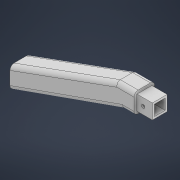
# Autodesk Inventor part: Fahrwerk_rocker_vorne
Saved by Autodesk Inventor 2021 (Build 250183000, 183)
## iProperties
Created: 2020-12-29
Part Number: Fahrwerk_rocker_vorne
Material: Generisch
Document SubType Name: Modeling
Designer: laure
Density: 1 g/cm^3
Appearance: Vorgabe
Author: laure
## iProperties of the stored document _3D-Druck.ipt
Created: 2020-12-30
Part Number: _3D-Druck
Material: Generisch
Document SubType Name: Modeling
Designer: laure
Density: 1 g/cm^3
Appearance: Vorgabe
Author: laure
Autodesk Inventor part; units mm, degrees
ref_plane "YZ Plane" through (0, 0, 0) normal (1, 0, 0) x (0, 1, 0)
ref_plane "XZ Plane" through (0, 0, 0) normal (0, 1, 0) x (-1, 0, 0)
ref_plane "XY Plane" through (0, 0, 0) normal (0, 0, 1) x (1, 0, 0)
sketch "Skizze1" plane through (0, 0, 0) normal (0, 0, 1) x (1, 0, 0)
  line L0 (4.7064, 3.5044) -> (-12.7276, 3.5044)
  line L1 (-12.7276, 3.5044) -> (-116.0937, -34.1178)
  line L2 (4.7064, 3.5044) -> (4.7064, -16.4956)
  line L3 (4.7064, -16.4956) -> (-6.4216, -16.4956)
  line L4 (-6.4216, -16.4956) -> (-116.0937, -55.3341)
  line L5 (-116.0937, -34.1178) -> (-116.0937, -55.4014)
  line L6 (0, 15.2855) -> (0, -67.1826) projected
  line L7 (-140.2538, 0) -> (28.8665, 0) projected
  point P0 (0, 0)
  dimension "d0" = 17.434
  dimension "d1" = 110
  dimension "d4" = 20
  dimension "d5" = 11.128
  dimension "d38" = 4.7065
  dimension "d39" = 16.4956
  dimension "d40" = 20
  dimension "d44" = 160.499
  constraints: 12 end point, 2 vertical, 1 horizontal, 1 parallel, 1 point on line
  measures "d0" distance of L0.start L0.end
  measures "d1" distance of L0.end L1.end
  measures "d4" distance of L0.start L2.end
  measures "d5" distance of L2.end L3.end
  measures "d38" distance from line of point (0, 0) L2
  measures "d39" distance from line of point (0, 0) L3
  measures "d40" angle of L1 L0
  measures "d44" angle of L3 L4
ref_plane "Arbeitsebene2" through (4.7064, -12.4956, -10) normal (1, 0, 0) x (0, 0, -1)
sketch "Skizze3" plane through (4.7064, -12.4956, -10) normal (1, 0, 0) x (0, 0, -1)
  line L0 (-3, -65.9356) -> (-3, 0) projected
  line L1 (-17.2, 13.2) -> (-2.8, 13.2)
  line L2 (-2.8, 13.2) -> (-2.8, -1.2)
  line L3 (-2.8, -1.2) -> (-17.2, -1.2)
  line L4 (-17.2, -1.2) -> (-17.2, 13.2)
  line L5 (-4.8, 11.2) -> (-15.2, 11.2)
  line L6 (-15.2, 11.2) -> (-15.2, 0.8)
  line L7 (-15.2, 0.8) -> (-4.8, 0.8)
  line L8 (-4.8, 0.8) -> (-4.8, 11.2)
  line L9 (-2.8, -1.2) -> (-17.2, -1.2) projected
  line L10 (-17.2, -1.2) -> (-17.2, 13.2) projected
  point P0 (-3, -1.2)
  point P1 (-3, 0)
  dimension "d13" = 14.4
  dimension "d14" = 14.4
  dimension "d15" = 2
  dimension "d31" = 0
  dimension "d32" = 0
  constraints: 16 end point, 4 parallel, 2 perpendicular, 1 horizontal, 3 other
  measures "d13" distance of L2.end L3.end
  measures "d14" distance of L1.end L2.end
  measures "d15" distance between parallel lines of L1 L5
  measures "d31" distance between parallel lines of L9 L3
  measures "d32" distance between parallel lines of L10 L4
extrude "Extrusion2" add sketch "Skizze3" along normal blind 15 and the other way blind 7.5
sketch "Skizze5" plane through (-2.7936, -13.6956, 7.2) normal (0, 0, 1) x (1, 0, 0)
  circle A0 centre (13.5, 7.2) radius 1.6
  line L0 (22.5, 14.4) -> (22.5, 0) projected
  line L1 (0, 0) -> (22.5, 0) projected
  dimension "d29" = 3.2
  dimension "d47" = 7.2
  dimension "d48" = 9
  constraints: 1 centre point
  measures "d29" diameter of A0
  measures "d47" distance from line of L1 A0.centre
  measures "d48" distance from line of L0 A0.centre
extrude "Extrusion4" cut sketch "Skizze5" against normal up to surface (14.4 mm away)
extrude "Extrusion5" add sketch "Skizze1" along normal mid plane 20
shell "Wandung2" thickness 2.6 removed faces 2 at (-116.0937, -48.262, 3.3333) at (4.7064, -4.7623, 1.7333)
fillet "Rundung5" radius 4 8 edges at (-64.4106, -15.3067, 10) (-64.4106, -15.3067, -10) (-61.2576, -35.9149, 10) (-61.2576, -35.9149, -10) (-0.8576, -16.4956, 10) (-4.0106, 3.5044, 10) (-4.0106, 3.5044, -10) (-0.8576, -16.4956, -10)
